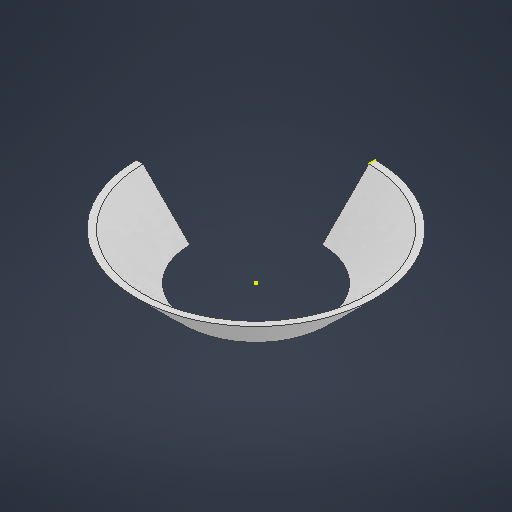
# Autodesk Inventor part: Holder at shooting
Saved by Autodesk Inventor 2026.2 (Build 302298010, 298A)
## iProperties
Created: 2026-04-19
Part Number: Holder at shooting
Material: Generic
Document SubType Name: Modeling
Designer: lenovo
Density: 1 g/cm^3
Appearance: Default
Author: lenovo
Autodesk Inventor part; units mm, degrees
ref_plane "YZ Plane" through (0, 0, 0) normal (1, 0, 0) x (0, 1, 0)
ref_plane "XZ Plane" through (0, 0, 0) normal (0, 1, 0) x (-1, 0, 0)
ref_plane "XY Plane" through (0, 0, 0) normal (0, 0, 1) x (1, 0, 0)
sketch "Sketch1" plane through (0, 0, 0) normal (0, 0, 1) x (1, 0, 0)
  line L0 (0, 0) -> (-14.1421, 14.1421)
  line L1 (0, 0) -> (20, 0) construction
  line L2 (-14.1421, 14.1421) -> (-16.1421, 14.1421)
  line L3 (-16.1421, 14.1421) -> (-12.4911, 10.4911)
  line L4 (20, 0) -> (20, 3.9234) construction
  line L5 (-12.4911, 10.4911) -> (-2, 0)
  line L6 (-2, 0) -> (0, 0)
  dimension "d1" = 20
  dimension "d2" = 135
  dimension "d3" = 2
  dimension "d5" = 2
  constraints: 14 end point, 3 horizontal, 1 equal length, 1 parallel, 1 vertical
  measures "d1" distance of L0.start L0.end
  measures "d2" angle of L1 L0
  measures "d3" distance of L0.end L2.end
  measures "d5" distance of L5.end L0.start
revolve "Revolution1" add sketch "Sketch1" angle 270 about axis through (20, 0, 0) along (0, 1, 0)
sketch "Sketch3" plane through (20, 14.1421, -36.1421) normal (-1, 0, 0) x (0, 0, 1)
  line L0 (2, 0) -> (0, 0) projected
  line L1 (0, 0) -> (0, -14.1421)
  line L2 (0, -14.1421) -> (2, -14.1421)
  line L3 (2, -14.1421) -> (2, 0)
  point P0 (36.1421, -14.1421)
  constraints: 6 end point, 2 perpendicular, 1 vertical
body "Solid1"
